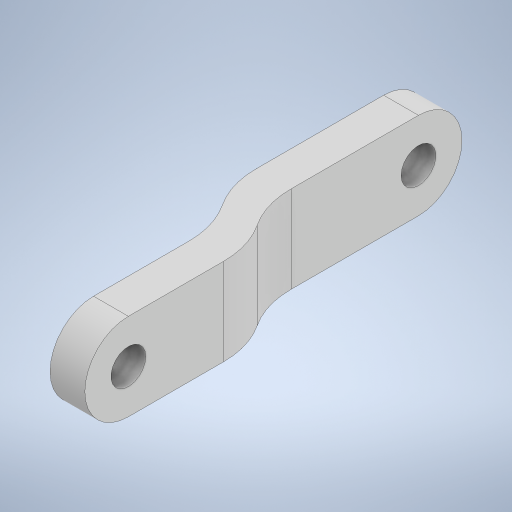
# Autodesk Inventor part: atividade_14A_uniao
Saved by Autodesk Inventor 2024.2 (Build 282272000, 272)
## iProperties
Created: 2024-03-04
Part Number: atividade_14A_uniao
Material: Generic
Document SubType Name: Modeling
Designer: 082220042
Density: 1 g/cm^3
Appearance: Default
Author: 082220042
Autodesk Inventor part; units mm, degrees
ref_plane "YZ Plane" through (0, 0, 0) normal (1, 0, 0) x (0, 1, 0)
ref_plane "XZ Plane" through (0, 0, 0) normal (0, 1, 0) x (-1, 0, 0)
ref_plane "XY Plane" through (0, 0, 0) normal (0, 0, 1) x (1, 0, 0)
sketch "Sketch1" plane through (0, 0, 0) normal (0, 1, 0) x (-1, 0, 0)
  line L0 (0, 0) -> (6, 0)
  line L1 (6, 0) -> (76, 0) construction
  line L2 (6, -70) -> (5, -70)
  line L3 (5, -70) -> (5, -51.6792)
  line L4 (5, -70) -> (11, -70)
  line L5 (11, -70) -> (11, -40.5)
  line L6 (5.0002, -40.5) -> (5, -40.5)
  line L7 (5, -40.5) -> (5, -70)
  line L8 (6, 0) -> (6, -23.9152)
  line L9 (0, -23.9152) -> (0, 0)
  arc A0 (-0.0017, -54.956) -> (0, -54.9555) centre (-3.9998, -40.4987) ccw
  arc A1 (-0.0017, -51.6807) -> (0, -51.6792) centre (-9.9998, -40.4987) ccw
  arc A2 (5, -40.5731) -> (2.5001, -32.2069) centre (-9.9998, -40.4987) ccw
  arc A3 (11, -40.5731) -> (8.5001, -32.2069) centre (-3.9998, -40.4987) ccw
  arc A4 (6, -23.9152) -> (8.5001, -32.2069) centre (21, -23.9152) ccw
  arc A5 (0, -23.9152) -> (2.5001, -32.2069) centre (15, -23.9152) ccw
  point P0 (6, -29.3181)
  point P1 (0, -29.3181)
  dimension "d0" = 6
  constraints: 20 end point, 15 point on circle, 6 centre point, 4 point on line, 4 tangent, 3 horizontal, 3 perpendicular, 2 parallel, 1 equal radius, 1 vertical
  measures "d0" distance of L0.start L0.end
extrude "Extrusion1" add sketch "Sketch1" along normal blind 15 contours L0 L8 A4 A0 A5 L9 | A0 L5 L3 L7 A1 A5 | L5 L4 L2 L3 A0
fillet "Fillet1" radius 7.5 4 edges at (-3, 0, 0) (-3, 15, 0) (-5.5, 15, -70) (-5.5, 0, -70)
sketch "Sketch3" plane through (0, 0, -23.9152) normal (1, 0, 0) x (0, 0, -1)
  circle A0 centre (-16.4152, 7.5) radius 3
  arc A1 (-16.4152, 15) -> (-16.4152, 0) centre (-16.4152, 7.5) ccw projected
  line L0 (-16.4152, 15) -> (0, 15) projected
  circle A2 centre (38.5848, 7.5) radius 3
  arc A3 (38.5848, 0) -> (38.5848, 15) centre (38.5848, 7.5) ccw projected
  line L1 (16.6579, 15) -> (38.5848, 15) projected
  point P0 (-23.9152, 0)
  point P1 (-23.9152, 7.5)
  point P2 (46.0848, 7.5)
  dimension "d15" = 6
  dimension "d16" = 7.5
  dimension "d17" = 7.5
  dimension "d18" = 6
  dimension "d19" = 7.5
  dimension "d20" = 7.5
  constraints: 2 centre point, 2 point on circle
  measures "d15" diameter of A0
  measures "d16" distance of point (-23.915, 7.5) A0.centre
  measures "d17" distance from line of L0 A0.centre
  measures "d18" diameter of A2
  measures "d19" distance of point (46.085, 7.5) A2.centre
  measures "d20" distance from line of L1 A2.centre
extrude "Extrusion2" cut sketch "Sketch3" against normal blind 15
body "Solid1"
